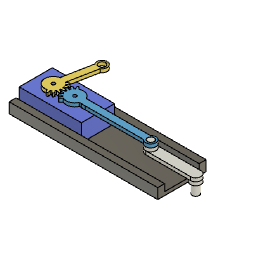
Rod Crank Gear Mechanism (Autodesk Fusion 360 design; units mm, degrees)
Autodesk Fusion 360 part; units mm, degrees
note: some values were not read from the file. Chosen so that the rebuilt part matches the saved one: which bodies a step acts on. Set by a fixed rule: which sketch regions a step uses.
sketch "holder" plane through (0, 0, 0) normal (0, 0, 1) x (1, 0, 0) in component "Holder"
  line L0 (-100, 35) -> (100, 35)
  line L1 (100, -35) -> (-100, -35)
  line L2 (-100, -35) -> (-100, 35)
  line L3 (-100, 25) -> (100, 25)
  line L4 (-100, -25) -> (100, -25)
  line L5 (100, 35) -> (110, 35)
  line L6 (110, -35) -> (100, -35)
  line L7 (100, -25) -> (110, -25)
  line L8 (100, 25) -> (110, 25)
  line L9 (110, 35) -> (115, 35)
  line L10 (115, 35) -> (115, -35)
  line L11 (115, -35) -> (110, -35)
  line L12 (110, 25) -> (115, 25)
  line L13 (110, -25) -> (115, -25)
  constraint horizontal L0
  constraint parallel L0 L1
  constraint coincident L2 L3.start
  constraint coincident L2 L4.start
  constraint perpendicular L9 L10
  constraint coincident L10 L12.end
  constraint perpendicular L10 L12
  constraint coincident L10 L13.end
  constraint perpendicular L10 L13
extrude "Extrude1" add sketch "holder" along normal blind 15 contours L0 L2 L3 L5 L8 L9 L10 L12 | L1 L2 L4 L6 L7 L10 L11 L13 makes body 1 at (-28.3333, -25, 5) makes body 2 at (-28.3333, 35, 5) in component "Holder"
extrude "Extrude2" add sketch "holder" along normal blind 5 contours L2 L3 L4 L7 L8 L10 L12 L13 bodies 1 2 in component "Holder"
sketch "slider" plane through (0, 0, 5) normal (0, 0, 1) x (-1, 0, 0) in component "Slider"
  line L0 (100, -25) -> (100, 25)
  line L1 (100, 25) -> (-115, 25)
  line L2 (-115, -25) -> (100, -25)
  line L3 (99, 24) -> (10, 24)
  line L4 (10, -24) -> (99, -24)
  line L5 (-100, -24) -> (-100, -24)
  line L6 (-100, 24) -> (-100, 24)
  line L7 (99, -24) -> (100, -24)
  line L8 (99, 24) -> (100, 24)
  line L9 (10, 0) -> (10, -24)
  line L10 (10, 0) -> (10, 25)
  line L11 (-115, 25) -> (-115, -25)
  constraint parallel L1 L3
  constraint parallel L2 L4
  constraint coincident L0 L7.end
  constraint perpendicular L0 L7
  constraint coincident L0 L8.end
  constraint perpendicular L0 L8
  constraint perpendicular L4 L9
  constraint coincident L1 L10.end
  constraint perpendicular L3 L10
  constraint coincident L10 L3.end
extrude "Extrude1'" add sketch "slider" along normal blind 25 separate body contours L0 L3 L4 L7 L8 L9 L10 makes body 3 in component "Slider"
sketch "crank suport" plane through (0, 0, 0) normal (0, 0, 1) x (1, 0, 0) in component "Crank"
  circle A0 centre (135, 0) radius 5
  dimension "d23" = 10
  measures "d23" diameter of A0
extrude "Extrude1''" add sketch "crank suport" along normal blind 15 separate body makes body 4 in component "Crank"
sketch "crank hand" plane through (0, 0, 15) normal (0, 0, 1) x (-1, 0, 0) in component "Crank"
  circle A0 centre (-135, 0) radius 5
  circle A1 centre (-135, 0) radius 7.5
  line L0 (-132.5, -7.5) -> (-135, -7.5)
  line L1 (-132.5, -7.5) -> (-70, -7.5)
  line L2 (-70, 7.5) -> (-135, 7.5)
  circle A2 centre (-70, 0) radius 7.5
  dimension "d26" = 15
  dimension "d27" = 15
  constraint concentric A0 A1
  constraint coincident A1 L0.end
  constraint tangent A1 L0
  constraint parallel L0 L1
  constraint coincident A1 L2.end
  constraint tangent A1 L2
  constraint coincident L1.end A2
  measures "d26" diameter of A1
  measures "d27" distance of L1.end L2.start
extrude "Extrude2'" add sketch "crank hand" along normal blind 10 contours A0 | A1 bodies 4 in component "Crank"
extrude "Extrude3" add sketch "crank hand" along normal blind 10 and the other way blind -5 contours A1 L0 L1 L2 A2 | A2 bodies 4 in component "Crank"
sketch "blue object" plane through (0, 0, 30) normal (0, 0, 1) x (-1, 0, 0) in component "blue thing with spur gear"
  line L0 (10, -24) -> (100, -24)
  line L1 (100, -24) -> (100, 24)
  line L2 (100, 24) -> (10, 24)
  line L3 (10, 24) -> (10, -24)
  circle A0 centre (-70, 0) radius 7.5
  circle A1 centre (-70, 0) radius 5
  line L4 (-53, -5) -> (-64.4098, -5)
  line L5 (-53, -5) -> (20, -5)
  line L6 (-60, 5) -> (-64.4098, 5)
  line L7 (-60, 5) -> (20, 5)
  line L8 (20, -5) -> (25.8579, -5)
  line L9 (20, 5) -> (25.8579, 5)
  circle A2 centre (40, 0) radius 2.5
  line L10 (25.8579, -5) -> (26.3893, -5)
  line L11 (25.8579, 5) -> (26.3893, 5)
  circle A3 centre (40, 0) radius 12.5
  arc A4 (50.0446, -13.0903) -> (48.2418, -9.398) centre (42.3606, -14.5557) ccw
  arc A5 (48.25, -14.2894) -> (50.0446, -13.0903) centre (40, 0) ccw
  arc A6 (45.5286, -11.2109) -> (48.25, -14.2894) centre (52.5443, -7.7511) ccw
  arc A7 (54.2894, -8.25) -> (51.2109, -5.5286) centre (47.7511, -12.5443) ccw
  arc A8 (53.0903, -10.0446) -> (54.2894, -8.25) centre (40, 0) ccw
  arc A9 (49.398, -8.2418) -> (53.0903, -10.0446) centre (54.5557, -2.3606) ccw
  arc A10 (56.3588, -2.1537) -> (52.4732, -0.8175) centre (51.9616, -8.6232) ccw
  arc A11 (55.9378, -4.2705) -> (56.3588, -2.1537) centre (40, 0) ccw
  arc A12 (51.8366, -4.018) -> (55.9378, -4.2705) centre (54.3511, 3.3893) ccw
  arc A13 (55.9378, 4.2705) -> (51.8366, 4.018) centre (54.3511, -3.3893) ccw
  arc A14 (56.3588, 2.1537) -> (55.9378, 4.2705) centre (40, 0) ccw
  arc A15 (52.4732, 0.8175) -> (56.3588, 2.1537) centre (51.9616, 8.6232) ccw
  arc A16 (53.0903, 10.0446) -> (49.398, 8.2418) centre (54.5557, 2.3606) ccw
  arc A17 (54.2894, 8.25) -> (53.0903, 10.0446) centre (40, 0) ccw
  arc A18 (51.2109, 5.5286) -> (54.2894, 8.25) centre (47.7511, 12.5443) ccw
  arc A19 (48.25, 14.2894) -> (45.5286, 11.2109) centre (52.5443, 7.7511) ccw
  arc A20 (50.0446, 13.0903) -> (48.25, 14.2894) centre (40, 0) ccw
  arc A21 (48.2418, 9.398) -> (50.0446, 13.0903) centre (42.3606, 14.5557) ccw
  line L12 (26.3893, -5) -> (28.5436, -5)
  line L13 (26.3893, 5) -> (28.5436, 5)
  dimension "d34" = 15
  dimension "d35" = 10
  dimension "d36" = 5
  constraint concentric A0 A1
  constraint coincident A0 L4.end
  constraint horizontal L4
  constraint perpendicular L3 L5
  constraint coincident A0 L6.end
  constraint parallel L4 L6
  constraint parallel L6 L7
  constraint horizontal L10
  constraint horizontal L11
  constraint coincident A3 L12.end
  constraint parallel L10 L12
  constraint coincident A3 L13.end
  constraint parallel L11 L13
  measures "d34" diameter of A0
  measures "d35" diameter of A1
  measures "d36" diameter of A2
extrude "Extrude1'''" add sketch "blue object" along normal blind 5 separate body contours L3 A0 L4 L5 L6 L7 | L3 L5 L7 L8 L9 L10 L11 A3 L12 L13 | A0 | A3 | A3 A4 A5 A6 | A3 A19 A20 A21 | A3 A7 A8 A9 | A3 A16 A17 A18 | A3 A10 A11 A12 | A3 A13 A14 A15 makes body 5 in component "blue thing with spur gear"
sketch "pin" plane through (0, 0, 25) normal (0, 0, 1) x (-1, 0, 0) in component "Crank"
  arc A0 (-135, 7.5) -> (-135, -7.5) centre (-135, 0) ccw
  line L0 (-135, -7.5) -> (-132.5, -7.5)
  line L1 (-132.5, -7.5) -> (-70, -7.5)
  arc A1 (-70, -7.5) -> (-70, 7.5) centre (-70, 0) ccw
  line L2 (-70, 7.5) -> (-135, 7.5)
  circle A2 centre (-70, 0) radius 7.5
  circle A3 centre (-70, 0) radius 4.7
extrude "Extrude4" add sketch "pin" along normal blind 10 contours A3 bodies 4 in component "Crank"
sketch "yellow object" plane through (0, 0, 30) normal (0, 0, 1) x (-1, 0, 0) in component "yellow thing with spur gear"
  line L0 (10, -24) -> (100, -24)
  line L1 (100, -24) -> (100, 24)
  line L2 (100, 24) -> (10, 24)
  line L3 (10, 24) -> (10, -24)
  circle A0 centre (70, 0) radius 2.5
  circle A1 centre (69.9381, -60.07) radius 5
  line L4 (74.9248, -13.638) -> (74.9436, -54.4848)
  arc A2 (64.9438, -54.4747) -> (74.9436, -54.4848) centre (69.9381, -60.07) ccw
  circle A3 centre (40, 0) radius 12.5
  arc A4 (54.0813, -4.3411) -> (58.1825, -4.0739) centre (55.6341, 3.4335) ccw
  arc A5 (57.523, -0.7586) -> (53.6318, -2.0812) centre (58.0416, -8.6698) ccw
  arc A6 (53.6318, -2.0812) -> (54.0813, -4.3411) centre (70, 0) ccw
  arc A7 (56.9543, -10.1024) -> (60.641, -8.2861) centre (55.4137, -2.3254) ccw
  arc A8 (58.7631, -5.4756) -> (55.6742, -8.1866) centre (62.2696, -12.5861) ccw
  arc A9 (55.6742, -8.1866) -> (56.9543, -10.1024) centre (70, 0) ccw
  arc A10 (61.8134, -14.3258) -> (64.5244, -11.2369) centre (57.4139, -7.7304) ccw
  arc A11 (61.7139, -9.359) -> (59.8976, -13.0457) centre (67.6746, -14.5863) ccw
  arc A12 (59.8976, -13.0457) -> (61.8134, -14.3258) centre (70, 0) ccw
  arc A13 (59.8976, 13.0457) -> (61.7139, 9.359) centre (67.6746, 14.5863) ccw
  arc A14 (64.5244, 11.2369) -> (61.8134, 14.3258) centre (57.4139, 7.7304) ccw
  arc A15 (61.8134, 14.3258) -> (59.8976, 13.0457) centre (70, 0) ccw
  arc A16 (55.6742, 8.1866) -> (58.7631, 5.4756) centre (62.2696, 12.5861) ccw
  arc A17 (60.641, 8.2861) -> (56.9543, 10.1024) centre (55.4137, 2.3254) ccw
  arc A18 (56.9543, 10.1024) -> (55.6742, 8.1866) centre (70, 0) ccw
  arc A19 (53.6318, 2.0812) -> (57.523, 0.7586) centre (58.0416, 8.6698) ccw
  arc A20 (58.1825, 4.0739) -> (54.0813, 4.3411) centre (55.6341, -3.4335) ccw
  arc A21 (54.0813, 4.3411) -> (53.6318, 2.0812) centre (70, 0) ccw
  arc A22 (74.0739, -11.8175) -> (64.5244, -11.2369) centre (70, 0) ccw
  line L5 (74.9248, -13.638) -> (74.9238, -11.4894)
  circle A23 centre (70, 0) radius 12.5
  line L6 (64.9438, -54.4747) -> (64.9438, -11.4317)
  dimension "d60" = 10
  dimension "d61" = 15
  dimension "d113" = 25
  dimension "d120" = 4
  dimension "d125" = 360
  constraint concentric A1 A2
  constraint concentric A6 A22
  constraint coincident A4.end A22
  constraint coincident A22 L5.end
  constraint parallel L4 L5
  constraint concentric A21 A23
  constraint coincident A10.end A23
  constraint vertical L6
  constraint coincident A23 L6.end
  measures "d60" diameter of A1
  measures "d61" diameter of A2
  measures "d113" diameter of A3
  measures "d120" distance of A6 A22
extrude "Extrude1''''" add sketch "yellow object" along normal blind 5 separate body contours L0 L4 A22 L5 A23 L6 | L0 L4 A2 L6 | A22 A23 | A10 A11 A12 A22 A23 | A7 A8 A9 A22 A23 | A13 A14 A15 A22 A23 | A4 A5 A6 A22 A23 | A16 A17 A18 A22 A23 | A19 A20 A21 A22 A23 makes body 6 in component "yellow thing with spur gear"
move_body "Move3" bodies 6 to x (0.979925, 0.199368, 0) y (-0.199368, 0.979925, 0) z (0, 0, 1) at (-2.7051, 13.9331, 0) in component "yellow thing with spur gear"
move_body "Move4" bodies 6 to x (0.92388, -0.382683, 0) y (0.382683, 0.92388, 0) z (0, 0, 1) at (-5.4187, -27.287, 0) in component "yellow thing with spur gear"
move_body "Move5" bodies 6 to x (1, 0, 0) y (0, 1, 0) z (0, 0, 1) at (0.3, 0, 0) in component "yellow thing with spur gear"
move_face "OffsetFaces1" offset 0.5 6 faces at (-54.5204, -0.8471, 31.6667) (-55.6803, -6.1516, 33.3333) (-58.668, -10.9852, 33.3333) (-65.4551, -15.5632, 31.6667) (-55.4593, 5.522, 31.6667) (-60.0373, 12.3091, 33.3333) on bodies 6 in component "yellow thing with spur gear"
move_face "OffsetFaces1'" offset 0.5 6 faces at (-49.8531, 13.235, 33.3333) (-54.1679, 8.457, 33.3333) (-55.9982, 4.0383, 31.6667) (-56.3258, -2.3914, 31.6667) (-54.1679, -8.457, 31.6667) (-49.8531, -13.235, 31.6667) on bodies 5 in component "blue thing with spur gear"
move_body "Move6" bodies 6 to x (1, 0, 0) y (0, 1, 0) z (0, 0, 1) at (0, -0.04, 0) in component "yellow thing with spur gear"
sketch "pins" plane through (0, 0, 30) normal (0, 0, 1) x (-1, 0, 0) in component "Slider"
  line L0 (10, -24) -> (100, -24)
  line L1 (100, -24) -> (100, 24)
  line L2 (100, 24) -> (10, 24)
  line L3 (10, 24) -> (10, -24)
  circle A0 centre (43.5, 0) radius 2.5
  circle A1 centre (74.5, 0.076) radius 2.2
  circle A2 centre (43.5, 0) radius 2.2
  dimension "d139" = -0.3
extrude "Extrude2''" add sketch "pins" along normal blind 5 contours A1 | A2 bodies 3 in component "Slider"
extrude "Extrude5" add sketch "pin" along normal blind 5 contours A1 A2 bodies 4 in component "Crank"
split "Split1" by plane through (0, 0, 25) normal (0, 0, 1) bodies 4 makes body 7 at (69.2532, 7.4627, 28.3333) in component "Crank"
split "Split2" by plane through (0, 0, 20) normal (0, 0, -1) bodies 4 makes body 8 at (139.9752, -0.4978, 10) in component "Crank"
component "Holder" placed x (1, 0, 0) y (0, 1, 0) z (0, 0, 1) at (0, 0, 0)
component "Slider" placed x (1, 0, 0) y (0, 1, 0) z (0, 0, 1) at (3.5089, 0, 0)
component "Crank" placed x (1, 0, 0) y (0, 1, 0) z (0, 0, 1) at (0, 0, 0)
component "blue thing with spur gear" placed x (1, 0, 0) y (0, 1, 0) z (0, 0, 1) at (0, 0, 0)
component "yellow thing with spur gear" placed x (1, 0, 0) y (0, 1, 0) z (0, 0, 1) at (0, 0, 0)
named bodies: "holder", "slider", "crank hand", "yellow object", "blue object", "crank pin", "crank stand"
